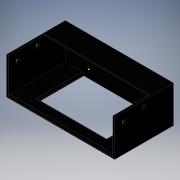
# Autodesk Inventor part: Bucket des 1
Saved by Autodesk Inventor 2016 (Build 200138000, 138)
## iProperties
Created: 2015-09-15
Part Number: Bucket des 1
Material: ABS Plastic
Document SubType Name: Modeling
Designer: tbloo
Density: 1.06 g/cm^3
Appearance: Smooth - White
Author: tbloo
Autodesk Inventor part; units mm, degrees
ref_plane "YZ Plane" through (0, 0, 0) normal (1, 0, 0) x (0, 1, 0)
ref_plane "XZ Plane" through (0, 0, 0) normal (0, 1, 0) x (-1, 0, 0)
ref_plane "XY Plane" through (0, 0, 0) normal (0, 0, 1) x (1, 0, 0)
sketch "Sketch1" plane through (0, 0, 0) normal (0, 1, 0) x (-1, 0, 0)
  point P0 (0, 0)
sketch "Sketch2" plane through (0, 0, 0) normal (0, 1, 0) x (-1, 0, 0)
  line L0 (-63.5, 112) -> (63.5, 112)
  line L1 (63.5, 112) -> (63.5, -112)
  line L2 (63.5, -112) -> (-63.5, -112)
  line L3 (-63.5, -112) -> (-63.5, 112)
  line L4 (-63.5, 112) -> (63.5, -112) construction
  line L5 (63.5, 112) -> (-63.5, -112) construction
  point P0 (0, 0)
  dimension "d0" = 127
  dimension "d1" = 224
  constraints: 12 end point, 2 midpoint, 2 parallel, 1 horizontal, 1 perpendicular
  measures "d0" distance of L1.end L2.end
  measures "d1" distance of L0.end L1.end
extrude "Extrusion1" add sketch "Sketch2" along normal blind 76.2
sketch "Sketch3" plane through (0, 76.2, 0) normal (0, 1, 0) x (1, 0, 0)
  line L0 (59.69, 107.95) -> (-59.69, 107.95)
  line L1 (-59.69, 107.95) -> (-59.69, -107.95)
  line L2 (-59.69, -107.95) -> (59.69, -107.95)
  line L3 (59.69, -107.95) -> (59.69, 107.95)
  line L4 (59.69, 107.95) -> (-59.69, -107.95) construction
  line L5 (-59.69, 107.95) -> (59.69, -107.95) construction
  point P0 (0, 0)
  dimension "d4" = 119.38
  dimension "d5" = 215.9
  constraints: 12 end point, 2 midpoint, 2 parallel, 1 horizontal, 1 perpendicular
  measures "d4" distance of L2.end L1.end
  measures "d5" distance of L1.end L0.end
extrude "Extrusion2" cut sketch "Sketch3" against normal blind 73.66
sketch "Sketch4" plane through (-59.69, 76.2, -107.95) normal (0, 0, 1) x (1, 0, 0)
  line L0 (119.38, 0) -> (119.38, -73.66) projected
  line L1 (119.38, 0) -> (0, 0)
  line L2 (0, 0) -> (0, -5.08)
  line L3 (0, -5.08) -> (119.38, -5.08)
  line L4 (119.38, -5.08) -> (119.38, 0)
  point P0 (59.69, -76.2)
  dimension "d8" = 5.08
  dimension "d11" = 119.38
  constraints: 8 end point, 2 parallel, 1 horizontal, 1 perpendicular
  measures "d8" distance of L2.end L1.end
  measures "d11" distance of L0.start L1.end
extrude "Extrusion3" add sketch "Sketch4" along normal blind 38.1
sketch "Sketch5" plane through (59.69, 76.2, 107.95) normal (0, 0, -1) x (-1, 0, 0)
  line L0 (0, 0) -> (119.38, 0)
  line L1 (119.38, 0) -> (119.38, -5.08)
  line L2 (119.38, -5.08) -> (0, -5.08)
  line L3 (0, -5.08) -> (0, 0)
  point P0 (59.69, -76.2)
  dimension "d12" = 5.08
  constraints: 8 end point, 2 parallel, 1 horizontal, 1 perpendicular
  measures "d12" distance of L0.end L1.end
extrude "Extrusion4" add sketch "Sketch5" along normal blind 38.1
sketch "Sketch7" plane through (63.5, 0, 112) normal (1, 0, 0) x (0, 0, -1)
  line L0 (224, 0) -> (0, 0) projected
  line L1 (224, 0) -> (224, 76.2) projected
  line L2 (0, 76.2) -> (224, 76.2) projected
  line L3 (0, 0) -> (0, 76.2) projected
  point P0 (112, 0)
extrude "Extrusion5" cut sketch "Sketch7" against normal blind 5.08
sketch "Sketch8" plane through (-59.69, 76.2, -69.85) normal (0, 0, 1) x (1, 0, 0)
  line L0 (0, -5.08) -> (118.11, -5.08) projected
  line L1 (118.11, 0) -> (0, 0) projected
  line L2 (118.11, -5.08) -> (92.71, -5.08)
  line L3 (92.71, -5.08) -> (92.71, 0)
  line L4 (92.71, 0) -> (118.11, 0)
  line L5 (118.11, 0) -> (118.11, -5.08)
  point P0 (59.69, -76.2)
  dimension "d17" = 25.4
  constraints: 8 end point, 2 parallel, 1 horizontal, 1 perpendicular, 1 point on line
  measures "d17" distance of L3.end L4.end
extrude "Extrusion6" add sketch "Sketch8" along normal blind 139.7
sketch "Sketch9" plane through (58.42, 0, 112) normal (1, 0, 0) x (0, 0, -1)
  line L0 (219.95, 2.54) -> (219.95, 71.12) projected
  line L1 (219.95, 2.54) -> (4.05, 2.54)
  line L2 (4.05, 2.54) -> (4.05, 0)
  line L3 (4.05, 0) -> (219.95, 0)
  line L4 (219.95, 0) -> (219.95, 2.54)
  point P0 (112, 0)
  constraints: 8 end point, 2 parallel, 1 horizontal, 1 perpendicular
extrude "Extrusion7" cut sketch "Sketch9" against normal blind 76.2
fillet "Fillet1" radius 3.175 1 edges at (58.42, 71.12, 0)
fillet "Fillet2" radius 3.175 1 edges at (-13.335, 71.12, -69.85)
fillet "Fillet3" radius 3.175 1 edges at (-13.335, 71.12, 69.85)
sketch "Sketch10" plane through (-63.5, 0, -112) normal (0, 0, -1) x (-1, 0, 0)
  circle A0 centre (-102.87, 19.05) radius 4
  point P0 (-63.5, 0)
  dimension "d27" = 8
  constraints: 1 centre point
  measures "d27" diameter of A0
hole "Hole1" at (39.37, 19.05, -112) direction (0, 0, 1) diameter 8 end through all
fillet "Fillet4" radius 3.175 1 edges at (33.02, 71.12, 0)
sketch "Sketch11" plane through (-63.5, 0, 112) normal (0, 0, 1) x (1, 0, 0)
  point P0 (63.5, 0)
  point P1 (60.96, 12.7)
hole "Hole2" at (-2.54, 12.7, 112) direction (0, 0, -1) diameter 8 end through all
body "Solid1"
